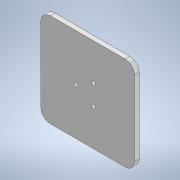
# Autodesk Inventor part: Tractor_Static_4
Saved by Autodesk Inventor 2022 (Build 260153070, 153G)
## iProperties
Created: 2022-03-05
Part Number: Tractor_Static_4
Material: Generic
Document SubType Name: Modeling
Designer: a laptop
Density: 1 g/cm^3
Appearance: Default
Author: a laptop
Autodesk Inventor part; units mm, degrees
ref_plane "YZ Plane" through (0, 0, 0) normal (1, 0, 0) x (0, 1, 0)
ref_plane "XZ Plane" through (0, 0, 0) normal (0, 1, 0) x (-1, 0, 0)
ref_plane "XY Plane" through (0, 0, 0) normal (0, 0, 1) x (1, 0, 0)
sketch "Sketch1" plane through (0, 0, 0) normal (0, 0, 1) x (1, 0, 0)
  circle A0 centre (0, 0) radius 14.925 construction
  circle A1 centre (12.4625, 21.5857) radius 4
  circle A2 centre (-24.925, 0) radius 4
  circle A3 centre (12.4625, -21.5857) radius 4
  line L0 (12.4625, -21.5857) -> (12.4625, 21.5857) construction
  line L1 (12.4625, 21.5857) -> (-24.925, 0) construction
  line L2 (-24.925, 0) -> (12.4625, -21.5857) construction
  line L3 (12.4625, 21.5857) -> (7.4625, 12.9254) construction
  line L4 (-14.925, 0) -> (-24.925, 0) construction
  line L5 (12.4625, -21.5857) -> (7.4625, -12.9254) construction
  line L6 (80, 100) -> (-80, 100)
  line L7 (-100, 80) -> (-100, -80)
  line L8 (-80, -100) -> (80, -100)
  line L9 (100, -80) -> (100, 80)
  arc A4 (100, 80) -> (80, 100) centre (80, 80) ccw
  arc A5 (-80, 100) -> (-100, 80) centre (-80, 80) ccw
  arc A6 (-100, -80) -> (-80, -100) centre (-80, -80) ccw
  arc A7 (80, -100) -> (100, -80) centre (80, -80) ccw
  circle A8 centre (0, 0) radius 5
  point P0 (100, 100)
  point P1 (-100, -100)
  point P2 (-100, 100)
  dimension "d0" = 29.85
  dimension "d1" = 8
  dimension "d2" = 10
  dimension "d3" = 200
  dimension "d4" = 200
  dimension "d5" = 100
  dimension "d6" = 100
  dimension "d7" = 20
  dimension "d10" = 10
  constraints: 20 end point, 11 point on circle, 9 centre point, 8 tangent, 6 point on line, 5 equal radius, 4 equal length, 3 line through centre, 2 coincident, 2 horizontal, 2 parallel, 1 perpendicular
  measures "d0" diameter of A0
  measures "d1" diameter of A1
  measures "d2" distance of L0.end L3.end
  measures "d3" distance of point (100, 100) point (-100, 100)
  measures "d4" distance of point (-100, 100) point (-100, -100)
  measures "d5" distance from line of L7 point (0, 0)
  measures "d6" distance from line of L6 point (0, 0)
  measures "d7" radius of A4
  measures "d10" diameter of A8
extrude "Extrusion1" add sketch "Sketch1" along normal blind 10
body "Solid1"
